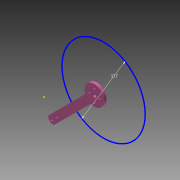
# Autodesk Inventor part: Arm2
Saved by Autodesk Inventor 2015 (Build 190159000, 159)
## iProperties
Created: 2017-01-13
Part Number: Arm2
Material: Generic
Document SubType Name: Modeling
Designer: Per
Density: 1 g/cm^3
Appearance: Pink
Author: Per
Autodesk Inventor part; units mm, degrees
ref_plane "YZ Plane" through (0, 0, 0) normal (1, 0, 0) x (0, 1, 0)
ref_plane "XZ Plane" through (0, 0, 0) normal (0, 1, 0) x (-1, 0, 0)
sketch "Sketch1" plane through (0, 0, 0) normal (0, 1, 0) x (-1, 0, 0)
  arc A0 (-76.1755, 50.0335) -> (-86.1582, 40.0508) centre (-90.5256, 54.4009) ccw
  circle A1 centre (-25.4718, -10.6529) radius 1.5
  line L0 (-24.7647, -15.6026) -> (-20.5221, -11.36)
  line L1 (-24.7647, -15.6026) -> (-29.0074, -15.6026)
  line L2 (-20.5221, -11.36) -> (-20.5221, -7.1174)
  circle A2 centre (-33.25, -2.8747) radius 1.5
  circle A3 centre (-90.5256, 44.9009) radius 1.5
  circle A4 centre (-98.5256, 54.4009) radius 1.5
  circle A5 centre (-90.5256, 63.9009) radius 1.5
  circle A6 centre (-82.5256, 54.4009) radius 1.5
  circle A7 centre (-90.5256, 54.4009) radius 3
  arc A8 (-76.1755, 50.0335) -> (-75.6764, 48.037) centre (-74.2622, 49.4512) ccw
  arc A9 (-84.1617, 39.5517) -> (-86.1582, 40.0508) centre (-85.5759, 38.1375) ccw
  line L3 (-75.6764, 48.037) -> (-71.4338, 43.7943)
  line L4 (-84.1617, 39.5517) -> (-79.919, 35.309)
  line L5 (-20.5221, -7.1174) -> (-71.4338, 43.7943)
  line L6 (-29.0074, -15.6026) -> (-79.919, 35.309)
  point P0 (0, 0)
  point P1 (-18.4008, -9.2387)
  point P2 (-76.5619, 48.9225)
  point P3 (-85.0472, 40.4372)
  point P4 (-26.886, -17.724)
  point P5 (-76.5619, 48.9225)
  dimension "d2" = 3
  dimension "d3" = 3
  dimension "d4" = 3
  dimension "d6" = 6
  dimension "d10" = 2
  constraints: 14 end point, 10 centre point, 8 point on circle, 2 point on line, 2 tangent, 1 coincident, 1 equal radius
  measures "d2" diameter of A3
  measures "d3" diameter of A4
  measures "d4" diameter of A5
  measures "d6" diameter of A7
  measures "d10" radius of A8
extrude "Extrusion3" add sketch "Sketch1" along normal blind 4
ref_plane "Motor Simulering" through (0, 14, 0) normal (0, 1, 0) x (1, 0, 0)
sketch "Propeller" plane through (0, 14, 0) normal (0, 1, 0) x (1, 0, 0)
  circle A0 centre (90.5256, -54.4009) radius 63.5
  point P0 (0, 0)
  dimension "d26" = 127
  constraints: 1 centre point, 1 coincident
  measures "d26" diameter of A0
body "Solid3"
